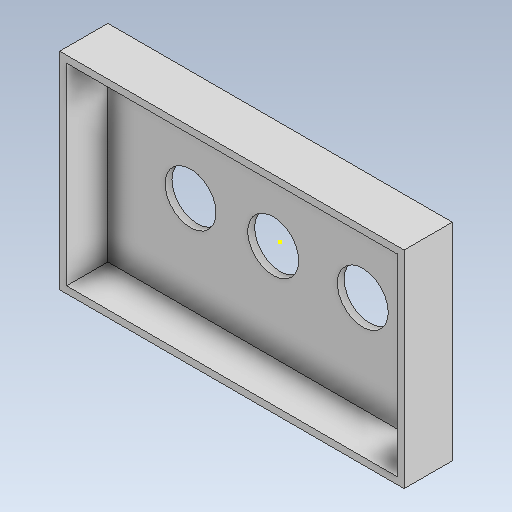
# Autodesk Inventor part: casing
Saved by Autodesk Inventor 2021 (Build 250183000, 183)
## iProperties
Created: 2023-06-22
Part Number: casing
Material: Generic
Document SubType Name: Modeling
Designer: mahmo
Density: 1 g/cm^3
Appearance: Default
Author: mahmo
Autodesk Inventor part; units mm, degrees
ref_plane "YZ Plane" through (0, 0, 0) normal (1, 0, 0) x (0, 1, 0)
ref_plane "XZ Plane" through (0, 0, 0) normal (0, 1, 0) x (-1, 0, 0)
ref_plane "XY Plane" through (0, 0, 0) normal (0, 0, 1) x (1, 0, 0)
sketch "Sketch1" plane through (0, 0, 0) normal (0, 0, 1) x (1, 0, 0)
  line L0 (-125, -75) -> (125, -75)
  line L1 (125, -75) -> (125, 75)
  line L2 (125, 75) -> (-125, 75)
  line L3 (-125, 75) -> (-125, -75)
  line L4 (-125, -75) -> (125, 75) construction
  line L5 (125, -75) -> (-125, 75) construction
  point P0 (0, 0)
  dimension "d0" = 250
  dimension "d1" = 150
  constraints: 12 end point, 2 midpoint, 2 parallel, 1 horizontal, 1 perpendicular
  measures "d0" distance of L2.end L1.end
  measures "d1" distance of L1.end L0.end
extrude "Extrusion1" add sketch "Sketch1" along normal blind 5
sketch "Sketch2" plane through (0, 0, 5) normal (0, 0, 1) x (1, 0, 0)
  line L0 (125, -75) -> (125, 75) projected
  line L1 (125, 75) -> (-125, 75) projected
  line L2 (-125, 75) -> (-125, -75) projected
  line L3 (-125, -75) -> (125, -75) projected
  line L4 (-120, 70) -> (120, 70)
  line L5 (120, 70) -> (120, -70)
  line L6 (120, -70) -> (-120, -70)
  line L7 (-120, -70) -> (-120, 70)
  point P0 (0, 0)
  dimension "d4" = 5
  constraints: 8 end point, 3 other
  measures "d4" distance between parallel lines of L1 L4
extrude "Extrusion2" add sketch "Sketch2" along normal blind 30
sketch "Sketch3" plane through (0, 0, 5) normal (0, 0, 1) x (1, 0, 0)
  line L0 (-120, 70) -> (-120, -70) projected
  line L1 (-120, -70) -> (120, -70) projected
  line L2 (120, -70) -> (120, 70) projected
  line L3 (120, 70) -> (-120, 70) projected
  circle A0 centre (0, 0) radius 18.5
  dimension "d8" = 37
  constraints: 1 centre point, 1 coincident
  measures "d8" diameter of A0
extrude "Extrusion3" cut sketch "Sketch3" against normal through all contours A0
sketch "Sketch4" plane through (0, 0, 0) normal (0, 0, -1) x (-1, 0, 0)
  circle A0 centre (-65, 0) radius 18.5
  circle A1 centre (60, 0) radius 18.5
  line L0 (125, 75) -> (125, -75) projected
  line L1 (-125, -75) -> (-125, 75) projected
  line L2 (125, -75) -> (-125, -75) projected
  point P0 (0, 0)
  dimension "d15" = 37
  dimension "d16" = 37
  dimension "d17" = 125
  dimension "d18" = 65
  dimension "d19" = 60
  dimension "d20" = 75
  constraints: 2 centre point
  measures "d15" diameter of A1
  measures "d16" diameter of A0
  measures "d17" distance of A0.centre A1.centre
  measures "d18" distance from line of L0 A1.centre
  measures "d19" distance from line of L1 A0.centre
  measures "d20" distance from line of L2 A0.centre
extrude "Extrusion4" cut sketch "Sketch4" against normal through all
sketch "Sketch5" plane through (0, 0, 0) normal (0, 0, -1) x (-1, 0, 0)
  point P0 (0, 0)
body "Solid1"
